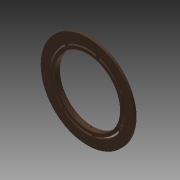
# Autodesk Inventor part: HandleTop01
Saved by Autodesk Inventor 2015 (Build 190159000, 159)
## iProperties
Created: 2016-08-08
Part Number: HandleTop01
Material: Generic
Document SubType Name: Modeling
Designer: spichelh
Density: 1 g/cm^3
Appearance: Default
Author: spichelh
Autodesk Inventor part; units mm, degrees
ref_plane "YZ Plane" through (0, 0, 0) normal (1, 0, 0) x (0, 1, 0)
ref_plane "Work Plane1" through (0, 0, 3) normal (0, 0, 1) x (1, 0, 0)
sketch "Sketch1" plane through (0, 0, 3) normal (0, 0, 1) x (1, 0, 0)
  circle A0 centre (0, 0) radius 74
  circle A1 centre (0, 0) radius 70
  dimension "d0" = 4
  dimension "d16" = 140
  constraints: 2 centre point, 2 coincident
  measures "d0" radial gap between concentric circles of A1 A0
  measures "d16" diameter of A1
extrude "Extrusion1" add sketch "Sketch1" against normal blind 11
sketch "Sketch2" plane through (0, 0, 3) normal (0, 0, 1) x (1, 0, 0)
  circle A0 centre (-48.5062, -131.4661) radius 70 projected
  circle A1 centre (0, 0) radius 74 projected
  point P0 (0, 0)
extrude "Extrusion2" [suppressed]
sketch "Sketch3" plane through (0, 0, -8) normal (0, 0, -1) x (-1, 0, 0)
  circle A0 centre (0, 0) radius 100
  circle A1 centre (0, 0) radius 74 projected
  arc A2 (55.1543, -55.1543) -> (78, 0) centre (0, 0) ccw construction
  arc A3 (56.215, -56.215) -> (79.5, 0) centre (0, 0) ccw
  arc A4 (54.0937, -54.0937) -> (76.5, 0) centre (0, 0) ccw
  arc A5 (54.0937, -54.0937) -> (56.215, -56.215) centre (55.1543, -55.1543) ccw
  arc A6 (79.5, 0) -> (76.5, 0) centre (78, 0) ccw
  line L0 (0, 0) -> (78.9092, -78.9092) construction
  line L1 (0, 0) -> (44.032, 0) construction
  line L2 (-12.8598, 72.874) -> (68.479, 72.874) construction
  arc A7 (77.5096, 8.7332) -> (48.6322, 60.9829) centre (0, 0) ccw construction
  arc A8 (79.0001, 8.9012) -> (49.5674, 62.1556) centre (0, 0) ccw
  arc A9 (76.019, 8.5653) -> (47.697, 59.8101) centre (0, 0) ccw
  arc A10 (76.019, 8.5653) -> (79.0001, 8.9012) centre (77.5096, 8.7332) ccw
  arc A11 (49.5674, 62.1556) -> (47.697, 59.8101) centre (48.6322, 60.9829) ccw
  arc A12 (41.4985, 66.0445) -> (-17.3566, 76.0444) centre (0, 0) ccw construction
  arc A13 (42.2966, 67.3146) -> (-17.6904, 77.5068) centre (0, 0) ccw
  arc A14 (40.7005, 64.7744) -> (-17.0229, 74.582) centre (0, 0) ccw
  arc A15 (40.7005, 64.7744) -> (42.2966, 67.3146) centre (41.4985, 66.0445) ccw
  arc A16 (-17.6904, 77.5068) -> (-17.0229, 74.582) centre (-17.3566, 76.0444) ccw
  arc A17 (-25.7618, 73.6229) -> (-70.2756, 33.8429) centre (0, 0) ccw construction
  arc A18 (-26.2572, 75.0387) -> (-71.627, 34.4938) centre (0, 0) ccw
  arc A19 (-25.2663, 72.2071) -> (-68.9241, 33.1921) centre (0, 0) ccw
  arc A20 (-25.2663, 72.2071) -> (-26.2572, 75.0387) centre (-25.7618, 73.6229) ccw
  arc A21 (-71.627, 34.4938) -> (-68.9241, 33.1921) centre (-70.2756, 33.8429) ccw
  arc A22 (-73.6229, 25.7618) -> (-70.2756, -33.8429) centre (0, 0) ccw construction
  arc A23 (-75.0387, 26.2572) -> (-71.627, -34.4938) centre (0, 0) ccw
  arc A24 (-72.2071, 25.2663) -> (-68.9241, -33.1921) centre (0, 0) ccw
  arc A25 (-72.2071, 25.2663) -> (-75.0387, 26.2572) centre (-73.6229, 25.7618) ccw
  arc A26 (-71.627, -34.4938) -> (-68.9241, -33.1921) centre (-70.2756, -33.8429) ccw
  arc A27 (-66.0445, -41.4985) -> (-17.3566, -76.0444) centre (0, 0) ccw construction
  arc A28 (-67.3146, -42.2966) -> (-17.6904, -77.5068) centre (0, 0) ccw
  arc A29 (-64.7744, -40.7005) -> (-17.0229, -74.582) centre (0, 0) ccw
  arc A30 (-64.7744, -40.7005) -> (-67.3146, -42.2966) centre (-66.0445, -41.4985) ccw
  arc A31 (-17.6904, -77.5068) -> (-17.0229, -74.582) centre (-17.3566, -76.0444) ccw
  arc A32 (-8.7332, -77.5096) -> (48.6322, -60.9829) centre (0, 0) ccw construction
  arc A33 (-8.9012, -79.0001) -> (49.5674, -62.1556) centre (0, 0) ccw
  arc A34 (-8.5653, -76.019) -> (47.697, -59.8101) centre (0, 0) ccw
  arc A35 (-8.5653, -76.019) -> (-8.9012, -79.0001) centre (-8.7332, -77.5096) ccw
  arc A36 (49.5674, -62.1556) -> (47.697, -59.8101) centre (48.6322, -60.9829) ccw
  point P0 (0, 0)
  point P1 (27.8096, 72.874)
  point P2 (-39.6362, 67.1786)
  point P3 (-77.2352, 10.8964)
  point P4 (-56.6745, -53.5911)
  point P5 (6.5633, -77.7234)
  point P6 (64.8587, -43.3284)
  point P7 (74.3142, 23.6938)
  dimension "d21" = 200
  dimension "d7" = 3
  dimension "d8" = 45
  dimension "d12" = 360
  dimension "d22" = 78
  constraints: 77 point on circle, 35 centre point, 6 end point, 4 tangent, 2 coincident, 2 horizontal, 2 point on line, 1 midpoint, 97 other
  measures "d7" diameter of A5
  measures "d8" angle of L1 L0
  measures "d22" distance of point (0, 0) A2.end
extrude "Extrusion3" add sketch "Sketch3" against normal blind 11
sketch "Sketch4" plane through (0, 0, -8) normal (0, 0, -1) x (-1, 0, 0)
  circle A0 centre (0, 0) radius 73.5
  circle A1 centre (0, 0) radius 105
  dimension "d17" = 147
  dimension "d18" = 210
  constraints: 2 centre point, 2 coincident
  measures "d17" diameter of A0
  measures "d18" diameter of A1
extrude "Extrusion4" cut sketch "Sketch4" against normal blind 6
sketch "Sketch5" plane through (0, 0, 3) normal (0, 0, 1) x (1, 0, 0)
  circle A0 centre (0, 0) radius 70 projected
  point P0 (0, -70)
  constraints: 1 vertical alignment, 1 other
ref_plane "Work Plane2" through (0, -70, 3) normal (0, -1, 0) x (1, 0, 0)
sketch "Sketch6" plane through (0, -70, 3) normal (0, -1, 0) x (1, 0, 0)
  circle A0 centre (0, -8) radius 1.5
  line L0 (-70, 0) -> (70, 0) projected
  line L1 (-73.5, -5) -> (73.5, -5) projected
  line L2 (-73.5, -11) -> (73.5, -11) projected
  line L3 (0, -7.7498) -> (0, -11) construction
  line L4 (70, -11) -> (-70, -11) construction
  point P0 (0, -3)
  dimension "d23" = 8
  dimension "d24" = 3
  constraints: 2 end point, 1 centre point, 1 midpoint, 1 point on line, 1 vertical
  measures "d23" distance from line of A0.centre L0
  measures "d24" diameter of A0
extrude "Extrusion5" cut sketch "Sketch6" along normal blind 6 and the other way blind 3
pattern_circular "Circular Pattern1" count 6 over 360 about axis through (0, 0, 3) along (0, 0, -1) of "Extrusion5"
body "Solid1"
